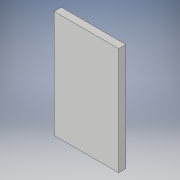
# Autodesk Inventor part: Halterplatte
Saved by Autodesk Inventor 2019 (Build 230136000, 136)
## iProperties
Created: 2021-05-01
Part Number: Halterplatte
Material: Generic
Document SubType Name: Modeling
Designer: Michael Sumper
Density: 1 g/cm^3
Appearance: Default
Author: Michael Sumper
Autodesk Inventor part; units mm, degrees
ref_plane "YZ Plane" through (0, 0, 0) normal (1, 0, 0) x (0, 1, 0)
ref_plane "XZ Plane" through (0, 0, 0) normal (0, 1, 0) x (-1, 0, 0)
ref_plane "XY Plane" through (0, 0, 0) normal (0, 0, 1) x (1, 0, 0)
sketch "Skizze1" plane through (0, 0, 0) normal (0, 0, 1) x (1, 0, 0)
  line L0 (-90, -150) -> (90, -150)
  line L1 (90, -150) -> (90, 150)
  line L2 (90, 150) -> (-90, 150)
  line L3 (-90, 150) -> (-90, -150)
  line L4 (-90, -150) -> (90, 150) construction
  line L5 (90, -150) -> (-90, 150) construction
  point P0 (0, 0)
  dimension "d0" = 180
  dimension "d1" = 300
  constraints: 12 end point, 2 midpoint, 2 parallel, 1 horizontal, 1 perpendicular
  measures "d0" distance of L2.end L1.end
  measures "d1" distance of L1.end L0.end
extrude "Extrusion1" add sketch "Skizze1" along normal blind 20
